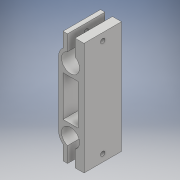
# Autodesk Inventor part: PiezaPeluda
Saved by Autodesk Inventor 2017 (Build 210142000, 142)
## iProperties
Part Number: PiezaPeluda
Material: Genérico
Document SubType Name: Modeling
Designer: osvaldo
Density: 1 g/cm^3
Appearance: Valor por defecto
Author: osvaldo
Autodesk Inventor part; units mm, degrees
ref_plane "YZ Plane" through (0, 0, 0) normal (1, 0, 0) x (0, 1, 0)
ref_plane "XZ Plane" through (0, 0, 0) normal (0, 1, 0) x (-1, 0, 0)
ref_plane "XY Plane" through (0, 0, 0) normal (0, 0, 1) x (1, 0, 0)
sketch "Boceto2" plane through (0, 0, 0) normal (0, 1, 0) x (-1, 0, 0)
  line L0 (-10, 37.5) -> (10, 37.5)
  line L1 (10, 37.5) -> (10, -37.5)
  line L2 (10, -37.5) -> (-10, -37.5)
  line L3 (-10, -37.5) -> (-10, 37.5)
  line L4 (-10, 37.5) -> (10, -37.5) construction
  line L5 (10, 37.5) -> (-10, -37.5) construction
  point P0 (0, 0)
  dimension "d10" = 20
  dimension "d11" = 75
  constraints: 12 end point, 2 midpoint, 2 parallel, 1 horizontal, 1 perpendicular
  measures "d10" distance of L1.end L2.end
  measures "d11" distance of L0.end L1.end
extrude "Extrusión1" add sketch "Boceto2" along normal blind 25
sketch "Boceto3" plane through (0, 25, 0) normal (0, 1, 0) x (1, 0, 0)
  line L0 (-10, -37.5) -> (10, -37.5) projected
  line L1 (10, -37.5) -> (10, 37.5) projected
  line L2 (10, 37.5) -> (-10, 37.5) projected
  line L3 (-10, 37.5) -> (-10, -37.5) projected
  arc A0 (3, -26.6962) -> (-2, -27.1569) centre (0, -21.5) ccw
  arc A1 (-8, -21.5) -> (-5, -27.745) centre (0, -21.5) ccw
  line L4 (-10, -37.5) -> (10, -37.5) projected
  line L5 (3, -37.5) -> (-2, -37.5)
  line L6 (3, -26.6962) -> (3, -37.5)
  line L7 (-5, -37.5) -> (-5, -27.745)
  line L8 (-8, -21.5) -> (-8, 21.5)
  line L9 (-5, -13.5) -> (5, -13.5)
  line L10 (-5, -13.5) -> (-5, 13.5)
  line L11 (7, 0) -> (10, 0)
  line L12 (-2, -37.5) -> (-2, -27.1569)
  line L13 (10, 0) -> (7, 0)
  arc A2 (-2, 27.1569) -> (3, 26.6962) centre (0, 21.5) ccw
  arc A3 (-5, 27.745) -> (-8, 21.5) centre (0, 21.5) ccw
  line L14 (3, 37.5) -> (-2, 37.5)
  line L15 (3, 26.6962) -> (3, 37.5)
  line L16 (-5, 37.5) -> (-5, 27.745)
  line L17 (-8, 21.5) -> (-8, 10)
  line L18 (-5, 13.5) -> (5, 13.5)
  line L19 (-5, 13.5) -> (-5, 10)
  line L20 (-2, 37.5) -> (-2, 27.1569)
  line L21 (5, -13.5) -> (5, 13.5)
  line L22 (-5, -37.5) -> (-10, -37.5)
  line L23 (-10, -37.5) -> (-10, 37.5)
  line L24 (10, 37.5) -> (-10, 37.5) projected
  line L25 (-10, 37.5) -> (-5, 37.5)
  point P0 (0, 0)
  point P1 (-8, -10)
  point P2 (-5, -10)
  dimension "d15" = 0
  dimension "d16" = 21.5
  dimension "d27" = 5
  dimension "d30" = 3
  dimension "d54" = 2
  dimension "d55" = 5
  dimension "d56" = 6
  dimension "d57" = 2
  dimension "d58" = 7
  dimension "d59" = 10
  constraints: 40 end point, 12 symmetric about line, 8 point on circle, 5 point on line, 4 centre point, 3 collinear, 3 perpendicular, 2 parallel, 1 horizontal, 1 midpoint, 1 tangent, 1 vertical, 2 other
  measures "d15" horizontal distance of point (0, 0) A0.centre
  measures "d16" distance of point (0, 0) A0.centre
  measures "d27" distance between parallel lines of L12 L6
  measures "d30" distance between parallel lines of L12 L7
  measures "d54" distance between parallel lines of L3 L8
  measures "d55" distance between parallel lines of L21 L1
  measures "d56" radius of A0
  measures "d57" radial gap between concentric circles of A0 A1
  measures "d58" distance between parallel lines of L1 L6
  measures "d59" distance between parallel lines of L21 L10
extrude "Extrusión3" cut sketch "Boceto3" against normal through all contours L12 A0 L6 L0 | L2 L15 A2 L20
extrude "Extrusión5" cut sketch "Boceto3" against normal through all contours L3 L2 L16 A3 L8 A1 L7 L0 | L10 L18 L21 L9
sketch "Boceto4" plane through (-8, 25, -21.5) normal (-1, 0, 0) x (0, 0, 1)
  line L0 (59, -25) -> (49.245, -25) projected
  line L1 (59, 0) -> (59, -25) projected
  line L2 (49.245, 0) -> (59, 0) projected
  line L3 (49.245, 0) -> (49.245, -25) projected
  line L4 (43, -25) -> (0, -25) projected
  line L5 (43, 0) -> (43, -25) projected
  line L6 (0, 0) -> (43, 0) projected
  line L7 (0, 0) -> (0, -25) projected
  line L8 (21.5, 0) -> (21.5, -25)
  line L9 (54.1225, -25) -> (54.1225, 0)
  line L10 (59, -12.5) -> (49.245, -12.5)
  point P0 (54.1225, -12.5)
  point P1 (54.1225, -12.5)
  point P2 (-11.1225, -12.5)
  constraints: 6 end point, 6 midpoint, 1 coincident, 1 symmetric about line, 1 vertical
hole "Agujero1" at (-8, 12.5, 32.6225) at (-8, 12.5, -32.6225) direction (1, 0, 0) diameter 3 end through all
sketch "Boceto5" plane through (0, 0, 0) normal (0, -1, 0) x (1, 0, 0)
  line L0 (-5, -27.745) -> (-5, -37.5) projected
  line L1 (-5, -37.5) -> (-2, -37.5) projected
  line L2 (-2, -37.5) -> (-2, -27.1569) projected
  arc A0 (3, -26.6962) -> (-2, -27.1569) centre (0, -21.5) ccw projected
  line L3 (3, -26.6962) -> (3, -37.5) projected
  line L4 (3, -37.5) -> (10, -37.5) projected
  line L5 (10, -37.5) -> (10, 37.5) projected
  line L6 (10, 37.5) -> (3, 37.5) projected
  line L7 (3, 37.5) -> (3, 26.6962) projected
  arc A1 (-2, 27.1569) -> (3, 26.6962) centre (0, 21.5) ccw projected
  line L8 (-2, 27.1569) -> (-2, 37.5) projected
  line L9 (-2, 37.5) -> (-5, 37.5) projected
  line L10 (-5, 37.5) -> (-5, 27.745) projected
  arc A2 (-5, 27.745) -> (-8, 21.5) centre (0, 21.5) ccw projected
  line L11 (-8, 21.5) -> (-8, -21.5) projected
  arc A3 (-8, -21.5) -> (-5, -27.745) centre (0, -21.5) ccw projected
  line L12 (5, 13.5) -> (5, -13.5) projected
  line L13 (5, -13.5) -> (-5, -13.5) projected
  line L14 (-5, -13.5) -> (-5, 13.5) projected
  line L15 (-5, 13.5) -> (5, 13.5) projected
  line L16 (6, -21.5) -> (6, 21.5)
  arc A4 (-2, 27.1569) -> (3, 26.6962) centre (0, 21.5) ccw projected
  arc A5 (3, -26.6962) -> (-2, -27.1569) centre (0, -21.5) ccw projected
  line L17 (9, 37.5) -> (9, -37.5)
  point P0 (0, 0)
  dimension "d60" = 3
  constraints: 4 end point, 2 point on circle, 2 point on line, 1 perpendicular, 1 tangent, 1 vertical
  measures "d60" distance between parallel lines of L16 L17
extrude "Extrusión6" cut sketch "Boceto5" against normal through all contours L17 L6 L5 L4
equation "\"d10\" = 20 * scale"
equation "\"d11\" = 75 * scale"
equation "\"d12\" = 25 * scale"
equation "\"d16\" = 21.5 * scale"
equation "\"d27\" = 5 * scale"
equation "\"d30\" = 3 * scale"
equation "\"d54\" = 2 * scale"
equation "\"d55\" = 5 * scale"
equation "\"d56\" = 6 * scale"
equation "\"d57\" = 2 * scale"
equation "\"d58\" = 7 * scale"
equation "\"d59\" = 10 * scale"
equation "\"scale\" = 1"
